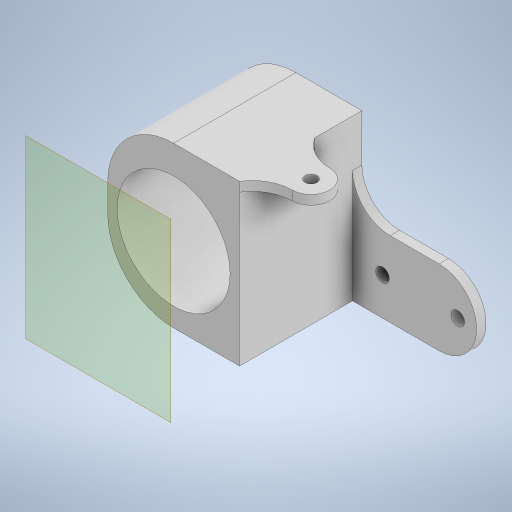
# Autodesk Inventor part: Motor Mount left
Saved by Autodesk Inventor 2024 (Build 280153000, 153)
## iProperties
Created: 2023-11-30
Part Number: Motor Mount left
Material: Generic
Document SubType Name: Modeling
Designer: CJ110
Density: 1 g/cm^3
Appearance: Default
Author: CJ110
## iProperties of the stored document Motor Mount right_3DPrint.ipt
Created: 2023-11-30
Part Number: Motor Mount right_3DPrint
Material: Generic
Document SubType Name: Modeling
Designer: CJ110
Density: 1 g/cm^3
Appearance: Default
Author: CJ110
Autodesk Inventor part; units mm, degrees
ref_plane "YZ Plane" through (0, 0, 0) normal (1, 0, 0) x (0, 1, 0)
ref_plane "XZ Plane" through (0, 0, 0) normal (0, 1, 0) x (-1, 0, 0)
ref_plane "XY Plane" through (0, 0, 0) normal (0, 0, 1) x (1, 0, 0)
sketch "Sketch1" plane through (0, 0, 0) normal (0, 1, 0) x (-1, 0, 0)
  line L0 (0, 0) -> (44.45, 0)
  line L1 (44.45, 0) -> (44.45, 50.8)
  line L2 (44.45, 50.8) -> (0, 50.8)
  line L3 (0, 50.8) -> (0, 0)
  circle A0 centre (22.225, 25.4) radius 19.05
  line L4 (44.45, 25.4) -> (0, 25.4) construction
  line L5 (22.225, 50.8) -> (22.225, 0) construction
  line L6 (44.45, 0) -> (44.45, -3.175)
  line L7 (44.45, -3.175) -> (0, -3.175)
  line L8 (0, -3.175) -> (0, 0)
  arc A1 (44.45, 28.575) -> (22.225, 50.8) centre (22.225, 28.575) ccw
  arc A2 (22.225, -3.175) -> (44.45, 19.05) centre (22.225, 19.05) ccw
  line L9 (22.225, -3.175) -> (22.225, 0)
  dimension "d1" = 38.1
  dimension "d2" = 50.8
  dimension "d22" = 44.45
  dimension "d37" = 3.175
  constraints: 20 end point, 6 midpoint, 4 perpendicular, 4 point on circle, 4 tangent, 3 centre point, 2 parallel, 2 point on line, 1 horizontal, 1 vertical
  measures "d1" diameter of A0
  measures "d2" distance of L5.start L5.end
  measures "d22" distance between parallel lines of L3 L1
  measures "d37" distance between parallel lines of L7 L0
extrude "Extrusion1" add sketch "Sketch1" against normal blind 38.1 contours L3 L2 A1 L1 A2 L0 | L0 L9 L7 L8 | L0 A2 L9
sketch "Sketch3" plane through (0, 0, 0) normal (0, 1, 0) x (1, 0, 0)
  line L0 (-44.45, -19.05) -> (-44.45, -28.575) projected
  line L1 (-22.225, -50.8) -> (0, -50.8) projected
  line L2 (0, -50.8) -> (0, 3.175) projected
  circle A0 centre (-22.225, -25.4) radius 19.05 projected
  circle A1 centre (-22.225, -25.4) radius 13.335
  circle A2 centre (-22.225, -9.906) radius 1.143
  circle A3 centre (-35.6432, -17.653) radius 1.143
  circle A4 centre (-35.6432, -33.147) radius 1.143
  circle A5 centre (-22.225, -40.894) radius 1.143
  circle A6 centre (-8.8068, -33.147) radius 1.143
  circle A7 centre (-8.8068, -17.653) radius 1.143
  line L3 (0, 3.175) -> (-22.225, 3.175) projected
  arc A8 (-22.225, 3.175) -> (-44.45, -19.05) centre (-22.225, -19.05) ccw projected
  arc A9 (-44.45, -28.575) -> (-22.225, -50.8) centre (-22.225, -28.575) ccw projected
  point P0 (0, 0)
  dimension "d6" = 26.67
  dimension "d7" = 2.286
  dimension "d8" = 15.494
  dimension "d11" = 360
  constraints: 7 centre point, 2 coincident, 1 vertical alignment, 13 other
  measures "d6" diameter of A1
  measures "d7" diameter of A2
  measures "d8" distance of point (-22.225, -25.4) A2.centre
extrude "Extrusion2" add sketch "Sketch3" along normal blind 3.175 contours A8 L3 L2 L1 A9 L0 | A0
sketch "Sketch4" plane through (0, 3.175, 0) normal (0, 1, 0) x (1, 0, 0)
  line L0 (-22.225, -50.8) -> (0, -50.8) projected
  line L1 (0, -50.8) -> (0, 3.175) projected
  line L2 (-44.45, -19.05) -> (-44.45, -28.575) projected
  circle A0 centre (-22.225, -25.4) radius 13.335 projected
  circle A1 centre (-22.225, -9.906) radius 1.143 projected
  circle A2 centre (-35.6432, -17.653) radius 1.143 projected
  circle A3 centre (-35.6432, -33.147) radius 1.143 projected
  circle A4 centre (-22.225, -40.894) radius 1.143 projected
  circle A5 centre (-8.8068, -33.147) radius 1.143 projected
  circle A6 centre (-8.8068, -17.653) radius 1.143 projected
  line L3 (0, -25.4) -> (41.91, -25.4)
  line L4 (41.91, -25.4) -> (41.91, -50.8)
  line L5 (41.91, -50.8) -> (0, -50.8)
  line L6 (0, -50.8) -> (0, -25.4)
  circle A7 centre (10.16, -38.1) radius 2.286
  circle A8 centre (35.56, -38.1) radius 2.286
  line L7 (0, -38.1) -> (41.91, -38.1) construction
  arc A9 (29.21, -50.8) -> (29.21, -25.4) centre (29.21, -38.1) ccw
  arc A10 (0, -12.7) -> (12.7, -25.4) centre (12.7, -12.7) ccw
  arc A11 (-22.225, 3.175) -> (-44.45, -19.05) centre (-22.225, -19.05) ccw projected
  arc A12 (-44.45, -28.575) -> (-22.225, -50.8) centre (-22.225, -28.575) ccw projected
  line L8 (0, 3.175) -> (-22.225, 3.175) projected
  point P0 (0, 0)
  point P1 (0, -50.8)
  dimension "d15" = 10.16
  dimension "d16" = 25.4
  dimension "d17" = 4.572
  dimension "d18" = 25.4
  dimension "d19" = 6.35
  dimension "d30" = 12.7
  constraints: 10 end point, 8 point on line, 5 point on circle, 4 centre point, 3 tangent, 2 midpoint, 2 parallel, 1 collinear, 1 equal radius, 1 horizontal, 1 perpendicular
  measures "d15" distance from line of L6 A7.centre
  measures "d16" distance of A7.centre A8.centre
  measures "d17" diameter of A8
  measures "d18" distance between parallel lines of L5 L3
  measures "d19" distance from line of L4 A8.centre
  measures "d30" distance from line of L1 A10.end
extrude "Extrusion3" add sketch "Sketch4" against normal blind 3.175 contours L1 L3 A9 L5 | L1 A10 L3
sketch "Sketch6" plane through (0, -38.1, -3.175) normal (0, 0, -1) x (-1, 0, 0)
  line L0 (0, 0) -> (0, 41.275) projected
  line L1 (44.45, 0) -> (0, 0) projected
  line L2 (0, 41.275) -> (44.45, 41.275) projected
  line L3 (0, 19.05) -> (-17.78, 19.05)
  line L4 (-17.78, 19.05) -> (-17.78, 6.35)
  line L5 (-17.78, 6.35) -> (0, 6.35)
  line L6 (0, 6.35) -> (0, 19.05)
  circle A0 centre (-11.43, 12.7) radius 2.032
  line L7 (0, 12.7) -> (-17.78, 12.7) construction
  circle A1 centre (-11.43, 12.7) radius 6.35
  arc A2 (0, 0) -> (-11.43, 6.35) centre (-11.43, -7.112) ccw
  line L8 (0, 0) -> (0, 41.275) projected
  arc A3 (-11.43, 19.05) -> (0, 25.4) centre (-11.43, 32.512) ccw
  line L9 (44.45, 41.275) -> (44.45, 0) projected
  point P0 (0, 38.1)
  point P1 (0, 25.4)
  dimension "d24" = 11.43
  dimension "d25" = 4.064
  dimension "d26" = 6.35
  dimension "d27" = 6.35
  dimension "d36" = 25.4
  constraints: 10 end point, 7 point on circle, 5 point on line, 4 centre point, 2 midpoint, 2 parallel, 2 tangent, 1 coincident, 1 equal radius, 1 horizontal, 1 perpendicular
  measures "d24" distance from line of L0 A0.centre
  measures "d25" diameter of A0
  measures "d26" distance from line of A0.centre L4
  measures "d27" distance from line of A0.centre L3
  measures "d36" vertical distance of point (0, 38.1) A1.centre
extrude "Extrusion4" add sketch "Sketch6" against normal blind 3.175 contours A2 L5 L0 | L5 A1 L3 L0 | A1 | L3 A3 L0
fillet "Fillet2" [suppressed]
ref_plane "Work Plane1" through (0, -63.5, 0) normal (0, -1, 0) x (1, 0, 0)
mirror "Mirror1" about plane through (0, -63.5, 0) normal (0, -1, 0) of "Extrusion4", "Extrusion3", "Extrusion2", "Extrusion1"
sketch "Sketch7" plane through (0, -63.5, 0) normal (0, -1, 0) x (1, 0, 0)
  line L0 (-66.3836, -28.6153) -> (65.8055, -28.6153)
  line L1 (65.8055, -28.6153) -> (65.8055, 56.7488)
  line L2 (65.8055, 56.7488) -> (-66.3836, 56.7488)
  line L3 (-66.3836, 56.7488) -> (-66.3836, -28.6153)
  point P0 (0, 0)
  constraints: 8 end point, 2 parallel, 1 horizontal, 1 perpendicular
extrude "Extrusion5" cut sketch "Sketch7" against normal through all
body "Solid1"
